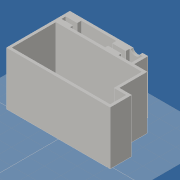
# Autodesk Inventor part: Erweiterung
Saved by Autodesk Inventor 2016 SP2 (Build 200236200, 236)
## iProperties
Created: 2018-07-08
Part Number: Erweiterung
Material: Generisch
Document SubType Name: Modeling
Designer: User
Density: 1 g/cm^3
Appearance: Vorgabe
Author: User
Autodesk Inventor part; units mm, degrees
ref_plane "YZ Plane" through (0, 0, 0) normal (1, 0, 0) x (0, 1, 0)
ref_plane "XZ Plane" through (0, 0, 0) normal (0, 1, 0) x (-1, 0, 0)
ref_plane "XY Plane" through (0, 0, 0) normal (0, 0, 1) x (1, 0, 0)
sketch "Skizze1" plane through (0, 0, 0) normal (0, 0, 1) x (1, 0, 0)
  line L0 (-60, 0) -> (60, 0)
  line L1 (60, 0) -> (60, 20)
  line L2 (60, 20) -> (45, 20)
  line L3 (45, 20) -> (45, 54)
  line L4 (-60, 41) -> (-60, 0)
  line L5 (-60, 41) -> (-60, 41)
  line L6 (-60, 54) -> (-60, 54)
  line L7 (-60, 54) -> (-60, 41)
  line L8 (29, 71) -> (29, 54)
  line L9 (29, 54) -> (45, 54)
  line L10 (-60, 54) -> (29, 54)
  line L11 (29, 54) -> (29, 57)
  line L12 (29, 57) -> (-60, 57)
  line L13 (-60, 57) -> (-60, 54)
  line L14 (29, 71) -> (-60, 71)
  line L15 (-60, 71) -> (-60, 54)
  line L16 (48, 23) -> (63, 23)
  line L17 (63, 23) -> (63, -3)
  line L18 (63, -3) -> (-63, -3)
  line L19 (-63, -3) -> (-63, 44)
  line L20 (-63, 44) -> (-63, 44)
  line L21 (-63, 44) -> (-63, 57)
  line L22 (-63, 57) -> (-63, 57)
  line L23 (-63, 57) -> (-63, 74)
  line L24 (-63, 74) -> (32, 74)
  line L25 (32, 74) -> (32, 57)
  line L26 (32, 57) -> (48, 57)
  line L27 (48, 57) -> (48, 23)
  line L28 (-60, 71) -> (-46, 71)
  line L29 (-46, 71) -> (-46, 66)
  line L30 (-46, 66) -> (-60, 66)
  line L31 (-60, 66) -> (-60, 71)
  line L32 (13, 71) -> (-3, 71)
  line L33 (-3, 71) -> (-3, 66)
  line L34 (-3, 66) -> (13, 66)
  line L35 (13, 66) -> (13, 71)
  line L36 (-60, 71) -> (-50, 71)
  line L37 (-50, 71) -> (-50, 66)
  line L38 (-50, 66) -> (-60, 66)
  line L39 (-60, 66) -> (-60, 71)
  line L40 (6, 71) -> (1, 71)
  line L41 (1, 71) -> (1, 66)
  line L42 (1, 66) -> (6, 66)
  line L43 (6, 66) -> (6, 71)
  line L44 (13, 71) -> (6, 71)
  line L45 (6, 71) -> (6, 66)
  line L46 (6, 66) -> (13, 66)
  line L47 (13, 66) -> (13, 71)
  line L48 (1, 71) -> (-3, 71)
  line L49 (-3, 71) -> (-3, 66)
  line L50 (-3, 66) -> (1, 66)
  line L51 (1, 66) -> (1, 71)
  line L52 (13, 57) -> (-3, 57)
  line L53 (-3, 57) -> (-3, 60.5)
  line L54 (-3, 60.5) -> (13, 60.5)
  line L55 (13, 60.5) -> (13, 57)
  line L56 (6, 60.5) -> (1, 60.5)
  line L57 (1, 60.5) -> (1, 57)
  line L58 (1, 57) -> (6, 57)
  line L59 (6, 57) -> (6, 60.5)
  line L60 (-60, 57) -> (-46, 57)
  line L61 (-46, 57) -> (-46, 60.5)
  line L62 (-46, 60.5) -> (-60, 60.5)
  line L63 (-60, 60.5) -> (-60, 57)
  line L64 (-50, 60.5) -> (-60, 60.5)
  line L65 (-60, 60.5) -> (-60, 57)
  line L66 (-60, 57) -> (-50, 57)
  line L67 (-50, 57) -> (-50, 60.5)
  line L68 (-60, 57) -> (29, 57)
  line L69 (29, 57) -> (29, 54)
  line L70 (29, 54) -> (-60, 54)
  line L71 (-60, 54) -> (-60, 57)
  point P0 (0, 0)
  point P1 (0, 0)
  point P2 (0, 0)
  point P3 (0, 0)
  dimension "d0" = 120
  dimension "d1" = 15
  dimension "d2" = 20
  dimension "d3" = 41
  dimension "d4" = 54
  dimension "d16" = 0
  dimension "d17" = 89
  dimension "d18" = 71
  dimension "d19" = 3
  dimension "d21" = 16
  dimension "d22" = 14
  dimension "d23" = 5
  dimension "d24" = 43
  dimension "d25" = 10
  dimension "d26" = 51
  dimension "d27" = 5
  dimension "d28" = 5.5
  dimension "d31" = 3
  dimension "d41" = 0
  constraints: 145 end point, 24 parallel, 22 perpendicular, 16 horizontal, 10 point on line, 9 collinear, 3 coincident, 1 midpoint, 1 vertical, 11 other
  measures "d0" distance between parallel lines of L1 L4
  measures "d1" distance between parallel lines of L1 L3
  measures "d2" distance between parallel lines of L0 L2
  measures "d3" distance between parallel lines of L0 L5
  measures "d4" distance between parallel lines of L0 L6
  measures "d16" distance between parallel lines of L7 L4
  measures "d17" distance of L8.start L14.end
  measures "d18" distance between parallel lines of L0 L14
  measures "d19" distance between parallel lines of L2 L16
  measures "d21" distance of L33.end L34.end
  measures "d22" distance of L29.end L30.end
  measures "d23" distance of L34.end L32.start
  measures "d24" distance between parallel lines of L29 L33
  measures "d25" distance between parallel lines of L15 L37
  measures "d26" distance between parallel lines of L37 L41
  measures "d27" distance between parallel lines of L41 L43
  measures "d28" distance between parallel lines of L54 L46
  measures "d31" distance between parallel lines of L10 L12
  measures "d41" distance between parallel lines of L23 L21
extrude "Extrusion1" add sketch "Skizze1" against normal blind 3 contours L4 L7 L10 L9 L3 L2 L1 L0 | L13 L12 L8 L10 | L15 L62 L67 L12 | L12 L55 L54 L53 L61 L62 L15 L30 L29 L14 L33 L34 L35 L8 | L67 L62 L61 L12 | L12 L59 L54 L55 | L15 L14 L37 L30 | L35 L34 L43 L14 | L12 L57 L54 L59 | L53 L54 L57 L12 | L37 L14 L29 L30 | L43 L34 L41 L14 | L41 L34 L33 L14 | L16 L17 L18 L19 L21 L23 L24 L25 L26 L27
extrude "Extrusion2" add sketch "Skizze1" along normal blind 62 contours L13 L12 L8 L10 | L15 L62 L67 L12 | L67 L62 L61 L12 | L12 L59 L54 L55 | L15 L14 L37 L30 | L35 L34 L43 L14 | L12 L57 L54 L59 | L53 L54 L57 L12 | L37 L14 L29 L30 | L43 L34 L41 L14 | L41 L34 L33 L14 | L16 L17 L18 L19 L21 L23 L24 L25 L26 L27
sketch "Skizze2" plane through (-63, 74, -3) normal (0, 1, 0) x (1, 0, 0)
  line L0 (95, -65) -> (95, 0) projected
  line L1 (95, -65) -> (0, -65) projected
  line L2 (92, -65) -> (76, -65) projected
  arc A0 (88.5, -65) -> (77, -65) centre (82.75, -66.7139) ccw
  line L3 (77, -65) -> (88.5, -65)
  point P0 (63, -3)
  dimension "d36" = 6
  dimension "d37" = 12.25
  dimension "d38" = 11.5
  constraints: 2 end point, 2 point on circle, 2 point on line, 1 centre point, 1 collinear
  measures "d36" radius of A0
  measures "d37" distance from line of L0 A0.centre
  measures "d38" distance of L3.end L3.start
extrude "Extrusion3" cut sketch "Skizze2" against normal up to surface (3 mm away)
